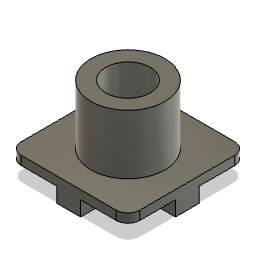
splicer_sample-fixation_013 (Autodesk Fusion 360 design; units mm, degrees)
Autodesk Fusion 360 part; units mm, degrees
sketch "Sketch1" plane through (0, 0, 0) normal (0, 1, 0) x (1, 0, 0)
  line L0 (20, -20) -> (-20, -20)
  line L1 (-20, -20) -> (-20, 20)
  line L2 (-20, 20) -> (20, 20)
  line L3 (20, 20) -> (20, -20)
  line L4 (20, -20) -> (-20, 20) construction
  line L5 (-20, -20) -> (20, 20) construction
  line L6 (-20, 4) -> (-15, 4)
  line L7 (-15, 4) -> (-15, -4)
  line L8 (-15, -4) -> (-20, -4)
  line L9 (-20, -4) -> (-20, 4)
  line L10 (-4, 20) -> (4, 20)
  line L11 (4, 20) -> (4, 15)
  line L12 (4, 15) -> (-4, 15)
  line L13 (-4, 15) -> (-4, 20)
  line L14 (20, 4) -> (15, 4)
  line L15 (15, 4) -> (15, -4)
  line L16 (15, -4) -> (20, -4)
  line L17 (20, -4) -> (20, 4)
  line L18 (-4, -20) -> (4, -20)
  line L19 (4, -20) -> (4, -15)
  line L20 (4, -15) -> (-4, -15)
  line L21 (-4, -15) -> (-4, -20)
  dimension "d1" = 40
  dimension "d2" = 40
  dimension "d3" = 5
  dimension "d4" = 8
  dimension "d5" = 16
  dimension "d6" = 5
  dimension "d7" = 16
  dimension "d8" = 8
  dimension "d9" = 5
  dimension "d10" = 5
  dimension "d11" = 8
  dimension "d12" = 8
  dimension "d13" = 16
  dimension "d14" = 16
  constraint horizontal L0
  constraint perpendicular L0 L1
  constraint parallel L0 L2
  constraint parallel L1 L3
  constraint coincident L4 origin
  constraint coincident L5 origin
  constraint horizontal L6
  constraint vertical L7
  constraint horizontal L8
  constraint vertical L9
  constraint coincident L1 L6.start
  constraint horizontal L10
  constraint vertical L11
  constraint horizontal L12
  constraint vertical L13
  constraint coincident L2 L10.start
  constraint horizontal L14
  constraint vertical L15
  constraint horizontal L16
  constraint vertical L17
  constraint coincident L3 L14.start
  constraint horizontal L18
  constraint vertical L19
  constraint horizontal L20
  constraint vertical L21
  constraint coincident L0 L18.start
  measures "d1" distance of L1.end L2.end
  measures "d2" distance of L0.end L1.end
  measures "d3" distance of L6.start L6.end
  measures "d4" distance of L6.start L8.end
  measures "d5" distance of L1.end L6.start
  measures "d6" distance of L10.start L12.end
  measures "d7" distance of L1.end L10.start
  measures "d8" distance of L11 L13
  measures "d9" distance of L18.start L20.end
  measures "d10" distance of L14.start L14.end
  measures "d11" distance of L14.end L15.end
  measures "d12" distance of L19.end L20.end
  measures "d13" distance of L1 L21
  measures "d14" distance of L0.start L16
extrude "Extrude1" add sketch "Sketch1" against normal blind 3 contours L0 L1 L2 L3 L6 L7 L8 L11 L12 L13 L14 L15 L16 L19 L20 L21
extrude "Extrude2" add sketch "Sketch1" against normal blind 8 contours L0 L18 L19 L20 L21 | L3 L14 L15 L16 L17 | L1 L6 L7 L8 L9 | L2 L10 L11 L12 L13
hole "Hole1" at (0, 0, 0) direction (0, -1, 0) diameter 9 depth 30 tip angle 118
fillet "Fillet1" radius 4 4 edges at (20, -1.5, -20) (-20, -1.5, -20) (20, -1.5, 20) (-20, -1.5, 20)
sketch "Sketch2" plane through (0, 0, 0) normal (0, 1, 0) x (-1, 0, 0)
  circle A0 centre (0, 0) radius 4.5
  arc A1 (20, 16) -> (16, 20) centre (16, 16) ccw
  line L0 (16, 20) -> (-16, 20)
  arc A2 (-16, 20) -> (-20, 16) centre (-16, 16) ccw
  line L1 (-20, 16) -> (-20, -16)
  arc A3 (-20, -16) -> (-16, -20) centre (-16, -16) ccw
  line L2 (-16, -20) -> (16, -20)
  arc A4 (16, -20) -> (20, -16) centre (16, -16) ccw
  line L3 (20, -16) -> (20, 16)
  circle A5 centre (0, 0) radius 12.5
  dimension "d24" = 25
  constraint concentric A0 A5
  measures "d24" diameter of A5
extrude "Extrude3" add sketch "Sketch2" along normal blind 20 contours A5
sketch "Sketch3" plane through (0, 20, 0) normal (0, 1, 0) x (-1, 0, 0)
  circle A0 centre (0, 0) radius 4.5
  circle A1 centre (0, 0) radius 12.5
hole "Hole2" at (0, 20, 0) direction (0, -1, 0) diameter 9 depth 40.942 tip angle 118 counterbore diameter 15 counterbore depth 20
equation "d6 = d3"
equation "d7 = d5"
equation "d8 = d4"
equation "d9 = d3"
equation "d10 = d3"
equation "d11 = d4"
equation "d12 = d4"
equation "d13 = d7"
equation "d14 = d7"
named bodies: "4040_fixation_base"
